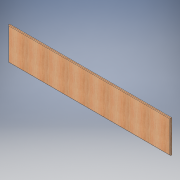
# Autodesk Inventor part: top
Saved by Autodesk Inventor 2016 (Build 200138000, 138)
## iProperties
Created: 2017-02-05
Part Number: top
Material: Wood (Birch)
Document SubType Name: Modeling
Designer: jwillauer
Density: 0.55 g/cm^3
Appearance: Birch - Natural Polished
Author: jwillauer
Autodesk Inventor part; units mm, degrees
ref_plane "YZ Plane" through (0, 0, 0) normal (1, 0, 0) x (0, 1, 0)
ref_plane "XZ Plane" through (0, 0, 0) normal (0, 1, 0) x (-1, 0, 0)
ref_plane "XY Plane" through (0, 0, 0) normal (0, 0, 1) x (1, 0, 0)
sketch "Sketch1" plane through (0, 0, 0) normal (0, 0, 1) x (1, 0, 0)
  line L0 (-1326.4924, 469.1885) -> (705.5076, 469.1885)
  line L1 (705.5076, 469.1885) -> (705.5076, 62.7885)
  line L2 (705.5076, 62.7885) -> (-1326.4924, 62.7885)
  line L3 (-1326.4924, 62.7885) -> (-1326.4924, 469.1885)
  point P0 (0, 0)
  dimension "d0" = 2032
  dimension "d1" = 406.4
  constraints: 8 end point, 2 parallel, 1 horizontal, 1 perpendicular
  measures "d0" distance of L0.start L0.end
  measures "d1" distance of L0.end L1.end
extrude "Extrusion1" add sketch "Sketch1" along normal blind 19.05
fillet "Fillet1" radius 6.35 4 edges at (-310.4924, 469.1885, 19.05) (705.5076, 265.9885, 19.05) (-310.4924, 62.7885, 19.05) (-1326.4924, 265.9885, 19.05)
body "Solid1"
